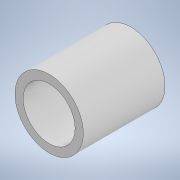
# Autodesk Inventor part: acople_2pulg
Saved by Autodesk Inventor 2021 (Build 250183000, 183)
## iProperties
Created: 2022-02-18
Part Number: acople_2pulg
Material: Genérico
Document SubType Name: Modeling
Designer: arthu
Density: 1 g/cm^3
Appearance: Valor por defecto
Author: arthu
Autodesk Inventor part; units mm, degrees
ref_plane "YZ Plane" through (0, 0, 0) normal (1, 0, 0) x (0, 1, 0)
ref_plane "XZ Plane" through (0, 0, 0) normal (0, 1, 0) x (-1, 0, 0)
ref_plane "XY Plane" through (0, 0, 0) normal (0, 0, 1) x (1, 0, 0)
sketch "Boceto1" plane through (0, 0, 0) normal (0, 0, 1) x (1, 0, 0)
  circle A0 centre (0, 0) radius 25.4
  circle A1 centre (0, 0) radius 33.4
  dimension "d0" = 50.8
  dimension "d1" = 8
  constraints: 2 centre point, 1 coincident
  measures "d0" diameter of A0
  measures "d1" radial gap between concentric circles of A0 A1
extrude "Extrusión1" add sketch "Boceto1" along normal blind 80
